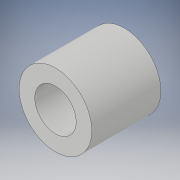
# Autodesk Inventor part: cylinderWrapVacuumInsulation
Saved by Autodesk Inventor 2018 (Build 220112000, 112)
## iProperties
Created: 2017-09-24
Part Number: cylinderWrapVacuumInsulation
Material: Generic
Document SubType Name: Modeling
Designer: Varun
Density: 1 g/cm^3
Appearance: Default
Author: Varun
Autodesk Inventor part; units mm, degrees
ref_plane "YZ Plane" through (0, 0, 0) normal (1, 0, 0) x (0, 1, 0)
ref_plane "XZ Plane" through (0, 0, 0) normal (0, 1, 0) x (-1, 0, 0)
ref_plane "XY Plane" through (0, 0, 0) normal (0, 0, 1) x (1, 0, 0)
sketch "Sketch1" plane through (0, 0, 0) normal (0, 0, 1) x (1, 0, 0)
  circle A0 centre (0, 0) radius 36.195
  circle A1 centre (0, 0) radius 63.5
  dimension "d0" = 72.39
  dimension "d1" = 127
  constraints: 2 centre point, 2 coincident
  measures "d0" diameter of A0
  measures "d1" diameter of A1
extrude "Extrusion1" add sketch "Sketch1" along normal blind 120.65
body "Solid1"
